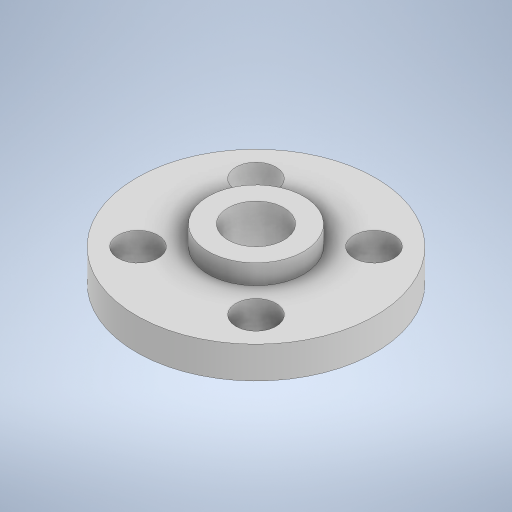
# Autodesk Inventor part: ANSI-B300-0.5S
Saved by Autodesk Inventor 2023 (Build 270158000, 158)
## iProperties
Company: Demo
Created: 2023-11-03
Part Number: ANSI-B300-0.5S
Material: Generic
Document SubType Name: Modeling
Designer: Admin
Density: 1 g/cm^3
Appearance: Default
Author: Admin
Autodesk Inventor part; units mm, degrees
ref_plane "YZ Plane" through (0, 0, 0) normal (1, 0, 0) x (0, 1, 0)
ref_plane "XZ Plane" through (0, 0, 0) normal (0, 1, 0) x (-1, 0, 0)
ref_plane "XY Plane" through (0, 0, 0) normal (0, 0, 1) x (1, 0, 0)
sketch "Sketch1" plane through (0, 0, 0) normal (0, 0, 1) x (1, 0, 0)
  line L0 (0, 0) -> (0, 22.1615) construction
  line L1 (-11.176, 22.1615) -> (-11.176, 0)
  line L2 (-11.176, 0) -> (-17.526, 0)
  line L3 (-17.526, 0) -> (-17.526, 1.5875)
  line L4 (-17.526, 1.5875) -> (-47.625, 1.5875)
  line L5 (-47.625, 1.5875) -> (-47.625, 14.2875)
  line L6 (-47.625, 14.2875) -> (-19.05, 14.2875)
  line L7 (-33.274, 14.2875) -> (-33.274, 1.5875) construction
  line L8 (-11.176, 22.1615) -> (-19.05, 22.1615)
  line L9 (-19.05, 22.1615) -> (-19.05, 14.2875)
  dimension "SB" = 22.352
  dimension "d1" = 1.5875
  dimension "SL" = 20.574
  dimension "Thickness" = 12.7
  dimension "R" = 35.052
  dimension "OD" = 95.25
  dimension "BC" = 66.548
  dimension "HB" = 38.1
  constraints: 20 end point, 6 vertical, 4 horizontal, 2 horizontal alignment, 2 point on line
  measures "SB" diameter of L1 L0
  measures "d1" distance between parallel lines of L2 L4
  measures "SL" distance from line of L1.start L4
  measures "Thickness" distance of L4.end L5.end
  measures "R" diameter of L3 L0
  measures "OD" diameter of L5 L0
  measures "BC" diameter of L7 L0
  measures "HB" diameter of L9 L0
revolve "Revolution1" add sketch "Sketch1" angle 360 about axis through (0, 0, 0) along (0, 1, 0)
sketch "Sketch2" plane through (0, 14.2875, 0) normal (0, 1, 0) x (1, 0, 0)
  line L0 (0, 0) -> (0, 47.625) construction
  circle A0 centre (0, 0) radius 47.625 projected
  line L1 (0, 0) -> (23.5283, 23.5283) construction
  dimension "d11" = 45
  dimension "d12" = 33.274
  constraints: 4 end point, 1 coincident, 1 vertical, 1 vertical alignment, 1 other
  measures "d11" angle of L1 L0
  measures "d12" distance of L1.start L1.end
hole "Hole1" at (23.5283, 14.2875, -23.5283) direction (0, -1, 0) diameter 16.002 depth 12.7
pattern_circular "Circular Pattern1" count 4 over 360 about axis through (0, -10, 0) along (0, 1, 0) of "Hole1"
equation "\"d12\" = 0.5 * BC"
body "Solid1"
